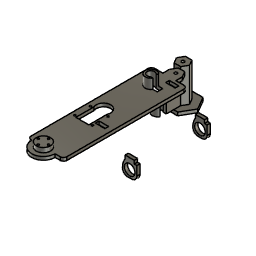
Arm Limb 2 Dynamixel v24 (Autodesk Fusion 360 design; units mm, degrees)
Autodesk Fusion 360 part; units mm, degrees
note: some values were not read from the file. Chosen so that the rebuilt part matches the saved one: which bodies a step acts on; which face or edge a step refers to. Set by a fixed rule: which sketch regions a step uses.
sketch "Sketch1" plane through (0, 0, 0) normal (0, 0, 1) x (1, 0, 0)
  circle A0 centre (25, 25) radius 1.5
  circle A1 centre (41, 25) radius 1.5
  circle A2 centre (33, 17) radius 1.5
  circle A3 centre (33, 33) radius 1.5
  circle A4 centre (33, 25) radius 18
  line L0 (15, 25) -> (51, 25)
  line L1 (51, 25) -> (51, 175)
  line L2 (51, 175) -> (15, 175)
  line L3 (15, 175) -> (15, 25)
  dimension "d1" = 3
  dimension "d2" = 3
  dimension "d3" = 3
  dimension "d4" = 3
  dimension "d5" = 36
  dimension "d6" = 150
  constraint horizontal L0
  constraint vertical L1
  constraint horizontal L2
  constraint vertical L3
  constraint coincident A4 L0.start
  measures "d1" diameter of A0
  measures "d2" diameter of A1
  measures "d3" diameter of A2
  measures "d4" diameter of A3
  measures "d5" distance of L0.start L0.end
  measures "d6" distance of L0.start L2.end
extrude "Extrude1" add sketch "Sketch1" along normal blind 5 contours A0 A1 A4 L0 | A0 A1 A4 L0 | A4 L1 L2 L3 makes body 1
sketch "Sketch4" plane through (0, 0, 0) normal (0, 0, 1) x (1, 0, 0)
  line L0 (50, 25) -> (70, 25)
  line L1 (70, 25) -> (70, 175)
  line L2 (70, 175) -> (50, 175)
  line L3 (50, 175) -> (50, 25)
  constraint horizontal L0
  constraint vertical L1
  constraint horizontal L2
  constraint vertical L3
extrude "Extrude3" add sketch "Sketch4" along normal blind 5 bodies 1
sketch "Sketch5" plane through (0, 0, 0) normal (0, 0, -1) x (1, 0, 0)
  line L0 (15, -175) -> (70, -175)
  line L1 (70, -175) -> (70, -25)
  line L2 (70, -25) -> (51, -25)
  arc A0 (51, -25) -> (15, -25) centre (33, -25) ccw
  line L3 (15, -25) -> (15, -175)
  circle A1 centre (33, -17) radius 1.5
  circle A2 centre (41, -25) radius 1.5
  circle A3 centre (25, -25) radius 1.5
  circle A4 centre (33, -33) radius 1.5
sketch "Sketch6" plane through (0, 0, 0) normal (0, 0, -1) x (1, 0, 0)
  line L0 (65.5, -170) -> (43.5, -170)
  line L1 (43.5, -170) -> (43.5, -165)
  line L2 (43.5, -165) -> (65.5, -165)
  line L3 (65.5, -165) -> (65.5, -170)
  line L4 (65.5, -62) -> (43.5, -62)
  line L5 (43.5, -62) -> (43.5, -57)
  line L6 (43.5, -57) -> (65.5, -57)
  line L7 (65.5, -57) -> (65.5, -62)
  dimension "d22" = 22
  dimension "d23" = 5
  dimension "d24" = 22
  dimension "d25" = 5
  constraint horizontal L0
  constraint vertical L1
  constraint horizontal L2
  constraint vertical L3
  constraint horizontal L4
  constraint vertical L5
  constraint horizontal L6
  constraint vertical L7
  measures "d22" distance of L0.start L0.end
  measures "d23" distance of L0.start L2.end
  measures "d24" distance of L4.start L4.end
  measures "d25" distance of L4.start L6.end
extrude "Extrude4" add sketch "Sketch6" along normal blind 22 bodies 1
sketch "Sketch7" plane through (0, 170, 0) normal (0, 1, 0) x (-1, 0, 0)
  line L0 (-43.5, 0) -> (-65.5, 0)
  line L1 (-65.5, 0) -> (-65.5, -22)
  line L2 (-65.5, -22) -> (-43.5, -22)
  line L3 (-43.5, -22) -> (-43.5, 0)
  circle A0 centre (-54.5, -11) radius 8.15
  dimension "d28" = 16.3
  measures "d28" diameter of A0
extrude "Extrude5" cut sketch "Sketch7" against normal blind 115 contours A0 bodies 1
fillet "Fillet1" radius 8 4 edges at (65.5, 167.5, -22) (43.5, 167.5, -22) (65.5, 59.5, -22) (43.5, 59.5, -22) on bodies 1
fillet "Fillet2" radius 5 3 edges at (70, 175, 2.5) (15, 175, 2.5) (70, 25, 2.5) on bodies 1
sketch "Sketch8" plane through (0, 0, 5) normal (0, 0, 1) x (-1, 0, 0)
  circle A0 centre (-33, -17) radius 1.5
  circle A1 centre (-41, -25) radius 1.5
  circle A2 centre (-25, -25) radius 1.5
  circle A3 centre (-33, -33) radius 1.5
  arc A4 (-65, -25) -> (-70, -30) centre (-65, -30) ccw
  line L0 (-70, -30) -> (-70, -170)
  arc A5 (-70, -170) -> (-65, -175) centre (-65, -170) ccw
  line L1 (-65, -175) -> (-20, -175)
  arc A6 (-20, -175) -> (-15, -170) centre (-20, -170) ccw
  line L2 (-15, -170) -> (-15, -25)
  arc A7 (-15, -25) -> (-51, -25) centre (-33, -25) ccw
  line L3 (-51, -25) -> (-65, -25)
  circle A8 centre (-39, -150) radius 5.75
  line L4 (-49.0301, -147.5429) -> (-43.0301, -147.5429)
  line L5 (-43.0301, -147.5429) -> (-43.0301, -152.5429)
  line L6 (-43.0301, -152.5429) -> (-49.0301, -152.5429)
  line L7 (-49.0301, -152.5429) -> (-49.0301, -147.5429)
  dimension "d35" = 11.5
  dimension "d42" = 6
  dimension "d43" = 5
  constraint horizontal L4
  constraint vertical L5
  constraint horizontal L6
  constraint vertical L7
  measures "d35" diameter of A8
  measures "d42" distance of L4.start L4.end
  measures "d43" distance of L4.start L6.end
extrude "Extrude6" cut sketch "Sketch8" against normal blind 5 contours A8 L4 L5 L6 | A8 L4 L5 L6 | A8 L4 L6 L7 bodies 1
sketch "Sketch9" plane through (0, 0, 5) normal (0, 0, 1) x (-1, 0, 0)
  arc A0 (-44.1572, -152.5429) -> (-44.1986, -147.5429) centre (-39, -150) ccw
  circle A1 centre (-33, -17) radius 1.5
  circle A2 centre (-41, -25) radius 1.5
  circle A3 centre (-25, -25) radius 1.5
  circle A4 centre (-33, -33) radius 1.5
  arc A5 (-65, -25) -> (-70, -30) centre (-65, -30) ccw
  line L0 (-70, -30) -> (-70, -170)
  arc A6 (-70, -170) -> (-65, -175) centre (-65, -170) ccw
  line L1 (-65, -175) -> (-20, -175)
  arc A7 (-20, -175) -> (-15, -170) centre (-20, -170) ccw
  line L2 (-15, -170) -> (-15, -25)
  arc A8 (-15, -25) -> (-51, -25) centre (-33, -25) ccw
  line L3 (-51, -25) -> (-65, -25)
  circle A9 centre (-39, -150) radius 8.6023
  line L4 (-49.0301, -147.5429) -> (-44.1986, -147.5429)
  line L5 (-44.1572, -152.5429) -> (-49.0301, -152.5429)
  line L6 (-49.0301, -152.5429) -> (-49.0301, -147.5429)
  constraint concentric A0 A9
extrude "Extrude7" add sketch "Sketch9" along normal blind 15 contours A0 A9 L4 L5 picked at (-45.6694, -153.7111) bodies 1
sketch "Sketch10" plane through (0, 0, 0) normal (0, 0, -1) x (1, 0, 0)
  line L0 (47.5, -170) -> (61.5, -170)
  line L1 (61.5, -170) -> (61.5, -165)
  line L2 (61.5, -165) -> (47.5, -165)
  line L3 (47.5, -165) -> (47.5, -170)
  line L4 (47.2, -170.3) -> (61.8, -170.3)
  line L5 (61.8, -170.3) -> (61.8, -164.7)
  line L6 (61.8, -164.7) -> (47.2, -164.7)
  line L7 (47.2, -164.7) -> (47.2, -170.3)
  line L8 (47.5, -62) -> (61.5, -62)
  line L9 (61.5, -62) -> (61.5, -57)
  line L10 (61.5, -57) -> (47.5, -57)
  line L11 (47.5, -57) -> (47.5, -62)
  line L12 (47.2, -62.3) -> (61.8, -62.3)
  line L13 (61.8, -62.3) -> (61.8, -56.7)
  line L14 (61.8, -56.7) -> (47.2, -56.7)
  line L15 (47.2, -56.7) -> (47.2, -62.3)
  dimension "d66" = 14.6
  dimension "d67" = 5.6
  constraint horizontal L0
  constraint vertical L1
  constraint horizontal L2
  constraint horizontal L4
  constraint vertical L5
  constraint horizontal L6
  constraint vertical L7
  constraint horizontal L8
  constraint vertical L9
  constraint horizontal L10
  constraint horizontal L12
  constraint vertical L13
  constraint horizontal L14
  constraint vertical L15
  measures "d66" distance of L5 L7
  measures "d67" distance of L4 L6
extrude "Extrude8" cut sketch "Sketch10" against normal blind 5 bodies 1
split "Split1" by plane through (0, 0, 0) normal (0, 0, 1) bodies 1 makes body 2 at (30.9251, 77.9076, 0) makes body 3 at (52.1667, 170, 1.6667) makes body 4 at (46.3905, 60.3333, -11.8115) makes body 5 at (52.1667, 60.3333, 5)
sketch "Sketch11" plane through (0, 0, 5) normal (0, 0, 1) x (-1, 0, 0)
  arc A0 (-45.7179, -152.5429) -> (-45.7439, -147.5429) centre (-37.5, -150) ccw
  line L0 (-45.7179, -152.5429) -> (-47.5301, -152.5429)
  line L1 (-47.5301, -152.5429) -> (-47.5301, -147.5429)
  line L2 (-47.5301, -147.5429) -> (-45.7439, -147.5429)
  circle A1 centre (-33, -17) radius 1.5
  circle A2 centre (-41, -25) radius 1.5
  circle A3 centre (-25, -25) radius 1.5
  circle A4 centre (-33, -33) radius 1.5
  arc A5 (-65, -25) -> (-70, -30) centre (-65, -30) ccw
  line L3 (-70, -30) -> (-70, -170)
  arc A6 (-70, -170) -> (-65, -175) centre (-65, -170) ccw
  line L4 (-65, -175) -> (-20, -175)
  arc A7 (-20, -175) -> (-15, -170) centre (-20, -170) ccw
  line L5 (-15, -170) -> (-15, -25)
  arc A8 (-15, -25) -> (-51, -25) centre (-33, -25) ccw
  line L6 (-51, -25) -> (-65, -25)
  circle A9 centre (-48, -75.3257) radius 1.5
  circle A10 centre (-21, -75.3257) radius 1.5
  circle A11 centre (-21, -51.3257) radius 1.5
  circle A12 centre (-48, -51.3257) radius 1.5
  line L7 (-47.2, -170.3) -> (-61.8, -170.3)
  line L8 (-61.8, -170.3) -> (-61.8, -164.7)
  line L9 (-61.8, -164.7) -> (-47.2, -164.7)
  line L10 (-47.2, -164.7) -> (-47.2, -170.3)
  line L11 (-47.2, -62.3) -> (-61.8, -62.3)
  line L12 (-61.8, -62.3) -> (-61.8, -56.7)
  line L13 (-61.8, -56.7) -> (-47.2, -56.7)
  line L14 (-47.2, -56.7) -> (-47.2, -62.3)
  circle A13 centre (-34.5, -81.8257) radius 11
  line L15 (-24.5, -49.3257) -> (-24.5, -77.2431)
  line L16 (-44.5, -49.3257) -> (-44.5, -77.2431)
  line L17 (-44.5, -49.3257) -> (-24.5, -49.3257)
  line L18 (-15, -175) -> (-15, -25)
  line L19 (-47.2, -170.3) -> (-61.8, -170.3)
  line L20 (-61.8, -170.3) -> (-61.8, -164.7)
  line L21 (-61.8, -164.7) -> (-47.2, -164.7)
  line L22 (-47.2, -164.7) -> (-47.2, -170.3)
  line L23 (-47.2, -62.3) -> (-61.8, -62.3)
  line L24 (-61.8, -62.3) -> (-61.8, -56.7)
  line L25 (-61.8, -56.7) -> (-47.2, -56.7)
  line L26 (-47.2, -56.7) -> (-47.2, -62.3)
  arc A14 (-47.2179, -152.5429) -> (-47.2439, -147.5429) centre (-39, -150) ccw
  line L27 (-47.2179, -152.5429) -> (-49.0301, -152.5429)
  line L28 (-49.0301, -152.5429) -> (-49.0301, -147.5429)
  line L29 (-49.0301, -147.5429) -> (-47.2439, -147.5429)
  circle A15 centre (-33, -17) radius 1.5
  circle A16 centre (-41, -25) radius 1.5
  circle A17 centre (-25, -25) radius 1.5
  circle A18 centre (-33, -33) radius 1.5
  arc A19 (-65, -25) -> (-70, -30) centre (-65, -30) ccw
  line L30 (-70, -30) -> (-70, -170)
  arc A20 (-70, -170) -> (-65, -175) centre (-65, -170) ccw
  line L31 (-65, -175) -> (-20, -175)
  arc A21 (-20, -175) -> (-15, -170) centre (-20, -170) ccw
  line L32 (-15, -170) -> (-15, -25)
  arc A22 (-15, -25) -> (-51, -25) centre (-33, -25) ccw
  line L33 (-51, -25) -> (-65, -25)
  dimension "d46" = 3
  dimension "d47" = 3
  dimension "d48" = 3
  dimension "d49" = 3
  dimension "d59" = 9.5
  dimension "d69" = 3.5
  dimension "d70" = 3.5
  dimension "d71" = 3.5
  dimension "d72" = 3.5
  constraint coincident A13 L15.end
  constraint vertical L15
  constraint coincident A13 L16.end
  constraint parallel L15 L16
  constraint perpendicular L16 L17
  measures "d46" diameter of A9
  measures "d47" diameter of A10
  measures "d48" diameter of A11
  measures "d49" diameter of A12
  measures "d59" distance of L5 L15
  measures "d69" distance of A10.centre L15
  measures "d70" distance of A9.centre L16
  measures "d71" distance of A12.centre L16
  measures "d72" distance of A11.centre L15
extrude "Extrude9" cut sketch "Sketch11" against normal blind 5 contours A9 | A10 | A11 | A12 | A13 | A13 L15 L16 L17 bodies 2
move_body "Move5" bodies 4 1 to x (1, 0, 0) y (0, 1, 0) z (0, 0, 1) at (0, 0, -25)
move_body "Move6" bodies 3 5 to x (1, 0, 0) y (0, 1, 0) z (0, 0, 1) at (0, 0, -25)
combine "Combine7" operation add target body 1 tool bodies 3
combine "Combine8" operation add target body 5 tool bodies 4
move_body "Move10" bodies 5 1 to x (1, 0, 0) y (0, 1, 0) z (0, 0, 1) at (40, 0, 0)
sketch "Sketch12" plane through (0, 0, 5) normal (0, 0, 1) x (-1, 0, 0)
  circle A0 centre (-48, -75.3257) radius 1.5
  circle A1 centre (-21, -75.3257) radius 1.5
  circle A2 centre (-48, -51.3257) radius 1.5
  circle A3 centre (-21, -51.3257) radius 1.5
  line L0 (-47.2, -170.3) -> (-61.8, -170.3)
  line L1 (-61.8, -170.3) -> (-61.8, -164.7)
  line L2 (-61.8, -164.7) -> (-47.2, -164.7)
  line L3 (-47.2, -164.7) -> (-47.2, -170.3)
  line L4 (-47.2, -62.3) -> (-61.8, -62.3)
  line L5 (-61.8, -62.3) -> (-61.8, -56.7)
  line L6 (-61.8, -56.7) -> (-47.2, -56.7)
  line L7 (-47.2, -56.7) -> (-47.2, -62.3)
  arc A4 (-47.2179, -152.5429) -> (-47.2439, -147.5429) centre (-39, -150) ccw
  line L8 (-47.2179, -152.5429) -> (-49.0301, -152.5429)
  line L9 (-49.0301, -152.5429) -> (-49.0301, -147.5429)
  line L10 (-49.0301, -147.5429) -> (-47.2439, -147.5429)
  circle A5 centre (-33, -17) radius 1.5
  circle A6 centre (-41, -25) radius 1.5
  circle A7 centre (-25, -25) radius 1.5
  circle A8 centre (-33, -33) radius 1.5
  arc A9 (-65, -25) -> (-70, -30) centre (-65, -30) ccw
  line L11 (-70, -30) -> (-70, -170)
  arc A10 (-70, -170) -> (-65, -175) centre (-65, -170) ccw
  line L12 (-65, -175) -> (-20, -175)
  arc A11 (-20, -175) -> (-15, -170) centre (-20, -170) ccw
  line L13 (-15, -170) -> (-15, -25)
  arc A12 (-15, -25) -> (-51, -25) centre (-33, -25) ccw
  line L14 (-51, -25) -> (-65, -25)
  circle A13 centre (-33, -25) radius 11
  line L15 (-44.5, -49.3257) -> (-24.5, -49.3257)
  line L16 (-24.5, -49.3257) -> (-24.5, -77.2431)
  line L17 (-44.5, -77.2431) -> (-44.5, -49.3257)
  arc A14 (-44.5, -77.2431) -> (-24.5, -77.2431) centre (-34.5, -81.8257) ccw
  dimension "d52" = 22
  constraint concentric A12 A13
  measures "d52" diameter of A13
extrude "Extrude10" add sketch "Sketch12" along normal blind 7 contours A13 bodies 2
move_body "Move7" bodies 2 to x (1, 0, 0) y (0, 1, 0) z (0, 0, 1) at (0, -45, 0)
split "Split2" by plane through (0, 0, 0) normal (0, 1, 0) bodies 2 makes body 6 at (60.2767, 81.6143, 0)
move_body "Move8" bodies 6 to x (1, 0, 0) y (0, 1, 0) z (0, 0, 1) at (0, 40, 0)
extrude "Extrude11" add 1 faces at (51.6667, 0, 1.6667) along direction (0, 1, 0) blind 40 on bodies 2 bodies 2 6
chamfer "Chamfer1" distance 4 angle 45 2 edges at (83.5, 59.5, -25) (83.5, 167.5, -25) on bodies 1 5
fillet "Fillet3" radius 25 2 edges at (83.5, 167.5, -29) (83.5, 59.5, -29) on bodies 1 5
sketch "Sketch16" plane through (0, -20, 0) normal (0, -1, 0) x (1, 0, 0)
  line L0 (65, 0) -> (65, 5)
  line L1 (65, 5) -> (51, 5)
  line L2 (51, 5) -> (51, 0)
  line L3 (51, 0) -> (65, 0)
extrude "Extrude12" cut 1 faces at (32.9626, -17.8319, 12) along direction (0, 0, -1) blind 30 on bodies 2 bodies 2
sketch "Sketch18" plane through (0, -20, 0) normal (0, -1, 0) x (1, 0, 0)
  line L0 (65, 0) -> (15, 0)
  line L1 (15, 0) -> (15, 5)
  line L2 (15, 5) -> (65, 5)
  line L3 (65, 5) -> (65, 0)
  constraint horizontal L0
  constraint vertical L1
  constraint horizontal L2
  constraint vertical L3
extrude "Extrude15" add sketch "Sketch18" against normal blind 20 bodies 2
extrude "Extrude16" cut sketch "Sketch18" along normal blind 23 bodies 2
sketch "Sketch19" plane through (0, 0, 5) normal (0, 0, 1) x (-1, 0, 0)
  arc A0 (-47.2179, -147.5429) -> (-47.2439, -142.5429) centre (-39, -145) ccw
  line L0 (-47.2179, -147.5429) -> (-49.0301, -147.5429)
  line L1 (-49.0301, -147.5429) -> (-49.0301, -142.5429)
  line L2 (-49.0301, -142.5429) -> (-47.2439, -142.5429)
  line L3 (-47.2, -57.3) -> (-61.8, -57.3)
  line L4 (-61.8, -57.3) -> (-61.8, -51.7)
  line L5 (-61.8, -51.7) -> (-47.2, -51.7)
  line L6 (-47.2, -51.7) -> (-47.2, -57.3)
  line L7 (-47.2, -165.3) -> (-61.8, -165.3)
  line L8 (-61.8, -165.3) -> (-61.8, -159.7)
  line L9 (-61.8, -159.7) -> (-47.2, -159.7)
  line L10 (-47.2, -159.7) -> (-47.2, -165.3)
  line L11 (-24.5, -44.3257) -> (-24.5, -72.2431)
  arc A1 (-44.5, -72.2431) -> (-24.5, -72.2431) centre (-34.5, -76.8257) ccw
  line L12 (-44.5, -72.2431) -> (-44.5, -44.3257)
  circle A2 centre (-21, -70.3257) radius 1.5
  circle A3 centre (-48, -70.3257) radius 1.5
  line L13 (-15, 20) -> (-65, 20)
  arc A4 (-65, 20) -> (-70, 15) centre (-65, 15) ccw
  line L14 (-70, 15) -> (-70, -165)
  arc A5 (-70, -165) -> (-65, -170) centre (-65, -165) ccw
  line L15 (-65, -170) -> (-20, -170)
  arc A6 (-20, -170) -> (-15, -165) centre (-20, -165) ccw
  line L16 (-15, -165) -> (-15, 20)
  line L17 (-39, -145) -> (-15, -145)
  line L18 (-15, -145) -> (-15, 20)
  line L19 (-15, 20) -> (-39, 20)
  line L20 (-39, 20) -> (-39, -145)
  circle A7 centre (-39, 20) radius 18
  circle A8 centre (-39, 20) radius 11
  circle A9 centre (-21, -46.3257) radius 1.5
  circle A10 centre (-48, -46.3257) radius 1.5
  line L21 (-44.5, -44.3257) -> (-24.5, -44.3257)
  dimension "d86" = 36
  dimension "d87" = 22
  constraint horizontal L17
  constraint vertical L18
  constraint horizontal L19
  constraint vertical L20
  constraint coincident L13.start L16.end
  constraint coincident A0.centre L17.start
  constraint coincident L19.end L20.start
  constraint concentric A7 A8
  measures "d86" diameter of A7
  measures "d87" diameter of A8
extrude "Extrude17" add sketch "Sketch19" along normal blind 7 contours L13 L19 L20 A8 | L13 L19 A8 | L13 L20 A8 bodies 2
extrude "Extrude18" add sketch "Sketch19" against normal blind 5 contours L13 L19 A7 A8 | L13 L19 A8 bodies 2
sketch "Sketch21" plane through (0, 0, 12) normal (0, 0, 1) x (-1, 0, 0)
  circle A0 centre (-39, 20) radius 11
  line L0 (-47, 12) -> (-31, 12)
  line L1 (-31, 12) -> (-31, 28)
  line L2 (-31, 28) -> (-47, 28)
  line L3 (-47, 28) -> (-47, 12)
  line L4 (-47, 12) -> (-31, 28) construction
  line L5 (-31, 12) -> (-47, 28) construction
  circle A1 centre (-39, 12) radius 1.5
  circle A2 centre (-47, 20) radius 1.5
  circle A3 centre (-39, 28) radius 1.5
  circle A4 centre (-31, 20) radius 1.5
  point P0 (-39, 20)
  dimension "d94" = 16
  dimension "d95" = 16
  dimension "d96" = 3
  dimension "d97" = 3
  dimension "d98" = 3
  dimension "d99" = 3
  constraint horizontal L0
  constraint perpendicular L0 L1
  constraint parallel L0 L2
  constraint parallel L1 L3
  constraint coincident L4 P0
  constraint coincident L5 P0
  constraint coincident P0 A0.centre
  constraint midpoint L0 A1.centre
  constraint midpoint L3 A2.centre
  constraint midpoint L2 A3.centre
  constraint midpoint L1 A4.centre
  measures "d94" distance of L1.end L2.end
  measures "d95" distance of L0.end L1.end
  measures "d96" diameter of A1
  measures "d97" diameter of A2
  measures "d98" diameter of A3
  measures "d99" diameter of A4
extrude "Extrude19" cut sketch "Sketch21" against normal blind 20 contours L1 A4 | L1 A4 | L2 A3 | L2 A3 | L0 A1 | L0 A1 | L3 A2 | L3 A2 bodies 2
fillet "Fillet4" radius 5 1 edges at (15, -20, 2.5) on bodies 2
extrude "Extrude20" cut 1 faces at (49.0301, 145.8762, 3.3333) along direction (1, 0, 0) blind 2 on bodies 2 bodies 2
sketch "Sketch23" plane through (0, 170, 0) normal (0, 1, 0) x (-1, 0, 0)
  line L0 (-20, 0) -> (-20, 5)
  line L1 (-20, 5) -> (-65, 5)
  line L2 (-65, 5) -> (-65, 0)
  line L3 (-65, 0) -> (-20, 0)
  line L4 (-32.5, 0) -> (-52.5, 0)
  line L5 (-52.5, 0) -> (-52.5, 5)
  line L6 (-52.5, 5) -> (-32.5, 5)
  line L7 (-32.5, 5) -> (-32.5, 0)
  line L8 (-32.5, 0) -> (-52.5, 5) construction
  line L9 (-52.5, 0) -> (-32.5, 5) construction
  point P0 (-42.5, 2.5)
  constraint horizontal L4
  constraint perpendicular L4 L5
  constraint parallel L4 L6
  constraint parallel L5 L7
  constraint coincident L8 P0
  constraint coincident L9 P0
  constraint coincident L3 L4.start
extrude "Extrude23" add sketch "Sketch23" along normal blind 20 contours L1 L3 L4 L5 L6 L7 bodies 2
sketch "Sketch24" plane through (0, 0, 0) normal (0, 0, -1) x (1, 0, 0)
  line L0 (51.0301, -147.5429) -> (44.1572, -147.5429)
  arc A0 (44.1986, -142.5429) -> (44.1572, -147.5429) centre (39, -145) ccw
  line L1 (44.1986, -142.5429) -> (51.0301, -142.5429)
  line L2 (51.0301, -142.5429) -> (51.0301, -147.5429)
  arc A1 (20, 20) -> (15, 15) centre (20, 15) ccw
  line L3 (15, 15) -> (15, -165)
  arc A2 (15, -165) -> (20, -170) centre (20, -165) ccw
  line L4 (20, -170) -> (32.5, -170)
  line L5 (32.5, -170) -> (32.5, -190)
  line L6 (32.5, -190) -> (52.5, -190)
  line L7 (52.5, -190) -> (52.5, -170)
  line L8 (52.5, -170) -> (65, -170)
  arc A3 (65, -170) -> (70, -165) centre (65, -165) ccw
  line L9 (70, -165) -> (70, 15)
  arc A4 (70, 15) -> (65, 20) centre (65, 15) ccw
  line L10 (65, 20) -> (57, 20)
  arc A5 (57, 20) -> (21, 20) centre (39, 20) ccw
  line L11 (21, 20) -> (20, 20)
  circle A6 centre (39, 28) radius 1.5
  circle A7 centre (31, 20) radius 1.5
  circle A8 centre (47, 20) radius 1.5
  circle A9 centre (39, 12) radius 1.5
  circle A10 centre (48, -70.3257) radius 1.5
  circle A11 centre (21, -70.3257) radius 1.5
  line L12 (24.5, -72.2431) -> (24.5, -44.3257)
  line L13 (24.5, -44.3257) -> (44.5, -44.3257)
  line L14 (44.5, -44.3257) -> (44.5, -72.2431)
  arc A12 (24.5, -72.2431) -> (44.5, -72.2431) centre (34.5, -76.8257) ccw
  circle A13 centre (48, -46.3257) radius 1.5
  circle A14 centre (21, -46.3257) radius 1.5
  line L15 (47.2, -165.3) -> (47.2, -159.7)
  line L16 (47.2, -159.7) -> (61.8, -159.7)
  line L17 (61.8, -159.7) -> (61.8, -165.3)
  line L18 (61.8, -165.3) -> (47.2, -165.3)
  line L19 (47.2, -57.3) -> (47.2, -51.7)
  line L20 (47.2, -51.7) -> (61.8, -51.7)
  line L21 (61.8, -51.7) -> (61.8, -57.3)
  line L22 (61.8, -57.3) -> (47.2, -57.3)
  line L23 (32.5, -180) -> (37.5, -188.6603)
  line L24 (37.5, -188.6603) -> (47.5, -188.6603)
  line L25 (47.5, -188.6603) -> (52.5, -180)
  line L26 (52.5, -180) -> (47.5, -171.3397)
  line L27 (47.5, -171.3397) -> (37.5, -171.3397)
  line L28 (37.5, -171.3397) -> (32.5, -180)
  point P0 (42.5, -180)
  constraint midpoint L5 L23.start
extrude "Extrude24" cut sketch "Sketch24" against normal blind 5 contours L5 L6 L7 L23 L24 L25 bodies 2
extrude "Extrude25" add sketch "Sketch24" along normal blind 52 contours L23 L24 L25 L26 L27 L28 bodies 2
sketch "Sketch25" plane through (0, 0, -52) normal (0, 0, -1) x (1, 0, 0)
  line L0 (37.5, -171.3397) -> (32.5, -180)
  line L1 (32.5, -180) -> (37.5, -188.6603)
  line L2 (37.5, -188.6603) -> (47.5, -188.6603)
  line L3 (47.5, -188.6603) -> (52.5, -180)
  line L4 (52.5, -180) -> (47.5, -171.3397)
  line L5 (47.5, -171.3397) -> (37.5, -171.3397)
  line L6 (65, -180) -> (53.75, -160.5144)
  line L7 (53.75, -160.5144) -> (31.25, -160.5144)
  line L8 (31.25, -160.5144) -> (20, -180)
  line L9 (20, -180) -> (31.25, -199.4856)
  line L10 (31.25, -199.4856) -> (53.75, -199.4856)
  line L11 (53.75, -199.4856) -> (65, -180)
  point P0 (42.5, -180)
extrude "Extrude26" add sketch "Sketch25" along normal blind 5 contours L0 L1 L2 L3 L4 L5 | L6 L7 L8 L9 L10 L11 bodies 2
sketch "Sketch26" plane through (0, 0, 5) normal (0, 0, 1) x (-1, 0, 0)
  circle A0 centre (-48, -70.3257) radius 1.5
  circle A1 centre (-21, -70.3257) radius 1.5
  line L0 (-24.5, -44.3257) -> (-24.5, -72.2431)
  arc A2 (-44.5, -72.2431) -> (-24.5, -72.2431) centre (-34.5, -76.8257) ccw
  line L1 (-44.5, -72.2431) -> (-44.5, -44.3257)
  line L2 (-44.5, -44.3257) -> (-24.5, -44.3257)
  circle A3 centre (-48, -46.3257) radius 1.5
  circle A4 centre (-21, -46.3257) radius 1.5
  line L3 (-47.2, -165.3) -> (-61.8, -165.3)
  line L4 (-61.8, -165.3) -> (-61.8, -159.7)
  line L5 (-61.8, -159.7) -> (-47.2, -159.7)
  line L6 (-47.2, -159.7) -> (-47.2, -165.3)
  line L7 (-47.2, -57.3) -> (-61.8, -57.3)
  line L8 (-61.8, -57.3) -> (-61.8, -51.7)
  line L9 (-61.8, -51.7) -> (-47.2, -51.7)
  line L10 (-47.2, -51.7) -> (-47.2, -57.3)
  line L11 (-47.2179, -147.5429) -> (-51.0301, -147.5429)
  line L12 (-51.0301, -147.5429) -> (-51.0301, -142.5429)
  line L13 (-51.0301, -142.5429) -> (-47.2439, -142.5429)
  arc A5 (-47.2179, -147.5429) -> (-47.2439, -142.5429) centre (-39, -145) ccw
  line L14 (-52.5, -180) -> (-47.5, -188.6603)
  line L15 (-47.5, -188.6603) -> (-37.5, -188.6603)
  line L16 (-37.5, -188.6603) -> (-32.5, -180)
  line L17 (-32.5, -180) -> (-32.5, -170)
  line L18 (-32.5, -170) -> (-20, -170)
  arc A6 (-20, -170) -> (-15, -165) centre (-20, -165) ccw
  line L19 (-15, -165) -> (-15, 15)
  arc A7 (-15, 15) -> (-20, 20) centre (-20, 15) ccw
  line L20 (-20, 20) -> (-21, 20)
  arc A8 (-21, 20) -> (-57, 20) centre (-39, 20) ccw
  line L21 (-57, 20) -> (-65, 20)
  arc A9 (-65, 20) -> (-70, 15) centre (-65, 15) ccw
  line L22 (-70, 15) -> (-70, -165)
  arc A10 (-70, -165) -> (-65, -170) centre (-65, -165) ccw
  line L23 (-65, -170) -> (-52.5, -170)
  line L24 (-52.5, -170) -> (-52.5, -180)
  circle A11 centre (-39, 20) radius 11
  circle A12 centre (-42.5, -180) radius 2.25
  dimension "d121" = 4.5
  measures "d121" diameter of A12
extrude "Extrude27" cut sketch "Sketch26" against normal blind 16 contours A12 bodies 2
extrude "Extrude28" add 1 faces at (45.6682, 148.7131, 20) along direction (0, 0, -1) blind 65 on bodies 2 bodies 2
sketch "Sketch29" plane through (0, 0, 0) normal (0, 0, -1) x (1, 0, 0)
  line L0 (47.2, -57.3) -> (47.2, -51.7)
  line L1 (47.2, -51.7) -> (61.8, -51.7)
  line L2 (61.8, -51.7) -> (61.8, -57.3)
  line L3 (61.8, -57.3) -> (47.2, -57.3)
  line L4 (47.2, -165.3) -> (47.2, -159.7)
  line L5 (47.2, -159.7) -> (61.8, -159.7)
  line L6 (61.8, -159.7) -> (61.8, -165.3)
  line L7 (61.8, -165.3) -> (47.2, -165.3)
  circle A0 centre (21, -46.3257) radius 1.5
  circle A1 centre (48, -46.3257) radius 1.5
  line L8 (24.5, -72.2431) -> (24.5, -44.3257)
  line L9 (24.5, -44.3257) -> (44.5, -44.3257)
  line L10 (44.5, -44.3257) -> (44.5, -72.2431)
  arc A2 (24.5, -72.2431) -> (44.5, -72.2431) centre (34.5, -76.8257) ccw
  circle A3 centre (21, -70.3257) radius 1.5
  circle A4 centre (48, -70.3257) radius 1.5
  circle A5 centre (39, 12) radius 1.5
  circle A6 centre (47, 20) radius 1.5
  circle A7 centre (31, 20) radius 1.5
  circle A8 centre (39, 28) radius 1.5
  arc A9 (47.2439, -142.5429) -> (47.2179, -147.5429) centre (39, -145) ccw
  line L11 (47.2439, -142.5429) -> (51.0301, -142.5429)
  line L12 (51.0301, -142.5429) -> (51.0301, -147.5429)
  line L13 (51.0301, -147.5429) -> (47.2179, -147.5429)
  line L14 (47.5, -171.3397) -> (52.5, -180)
  line L15 (52.5, -180) -> (52.5, -170)
  line L16 (52.5, -170) -> (65, -170)
  arc A10 (65, -170) -> (70, -165) centre (65, -165) ccw
  line L17 (70, -165) -> (70, 15)
  arc A11 (70, 15) -> (65, 20) centre (65, 15) ccw
  line L18 (65, 20) -> (57, 20)
  arc A12 (57, 20) -> (21, 20) centre (39, 20) ccw
  line L19 (21, 20) -> (20, 20)
  arc A13 (20, 20) -> (15, 15) centre (20, 15) ccw
  line L20 (15, 15) -> (15, -165)
  arc A14 (15, -165) -> (20, -170) centre (20, -165) ccw
  line L21 (20, -170) -> (32.5, -170)
  line L22 (32.5, -170) -> (32.5, -180)
  line L23 (32.5, -180) -> (37.5, -171.3397)
  line L24 (37.5, -171.3397) -> (47.5, -171.3397)
  circle A15 centre (39, -145) radius 8.6023
  circle A16 centre (39, -145) radius 5.7423
  constraint concentric A9 A15
  constraint concentric A9 A16
extrude "Extrude29" cut sketch "Sketch29" along normal blind 25 contours A9 A15 bodies 2 makes body 7 at (47.111, 142.1344, -38.3333)
move_body "Move11" bodies 7 to x (1, 0, 0) y (0, 1, 0) z (0, 0, 1) at (0, 0, -7)
sketch "Sketch30" plane through (0, 171.3397, 0) normal (0, -1, 0) x (1, 0, 0)
  line L0 (47.5, 0) -> (37.5, 0)
  line L1 (37.5, 0) -> (37.5, -52)
  line L2 (37.5, -52) -> (47.5, -52)
  line L3 (47.5, -52) -> (47.5, 0)
  line L4 (37.5, -32) -> (47.5, -32)
  line L5 (47.5, -32) -> (47.5, -52)
  line L6 (47.5, -52) -> (37.5, -52)
  line L7 (37.5, -52) -> (37.5, -32)
  constraint horizontal L4
  constraint vertical L5
  constraint horizontal L6
  constraint vertical L7
  constraint coincident L2.end L3.start
  constraint coincident L1 L4.start
extrude "Extrude30" add sketch "Sketch30" along normal blind 24 contours L1 L2 L3 L4 L5 L6 L7 bodies 2 7
extrude "Extrude31" cut sketch "Sketch29" along normal blind 50 contours A16 bodies 2
split "Split3" by plane through (0, 0, 0) normal (0, 0, 1) bodies 2 makes body 8 at (52.6946, 6.3874, 0)
move_body "Move9" bodies 2 to x (1, 0, 0) y (0, 1, 0) z (0, 0, 1) at (-15, 25.9808, 0)
sketch "Sketch31" plane through (0, 0, 5) normal (0, 0, 1) x (-1, 0, 0)
  circle A0 centre (-42.5, -180) radius 2.25
  circle A1 centre (-48, -70.3257) radius 1.5
  circle A2 centre (-21, -70.3257) radius 1.5
  line L0 (-24.5, -44.3257) -> (-24.5, -72.2431)
  arc A3 (-44.5, -72.2431) -> (-24.5, -72.2431) centre (-34.5, -76.8257) ccw
  line L1 (-44.5, -72.2431) -> (-44.5, -44.3257)
  line L2 (-44.5, -44.3257) -> (-24.5, -44.3257)
  circle A4 centre (-48, -46.3257) radius 1.5
  circle A5 centre (-21, -46.3257) radius 1.5
  line L3 (-47.2, -165.3) -> (-61.8, -165.3)
  line L4 (-61.8, -165.3) -> (-61.8, -159.7)
  line L5 (-61.8, -159.7) -> (-47.2, -159.7)
  line L6 (-47.2, -159.7) -> (-47.2, -165.3)
  line L7 (-47.2, -57.3) -> (-61.8, -57.3)
  line L8 (-61.8, -57.3) -> (-61.8, -51.7)
  line L9 (-61.8, -51.7) -> (-47.2, -51.7)
  line L10 (-47.2, -51.7) -> (-47.2, -57.3)
  line L11 (-47.2179, -147.5429) -> (-51.0301, -147.5429)
  line L12 (-51.0301, -147.5429) -> (-51.0301, -142.5429)
  line L13 (-51.0301, -142.5429) -> (-47.2439, -142.5429)
  arc A6 (-47.2179, -147.5429) -> (-47.2439, -142.5429) centre (-39, -145) ccw
  line L14 (-52.5, -180) -> (-47.5, -188.6603)
  line L15 (-47.5, -188.6603) -> (-37.5, -188.6603)
  line L16 (-37.5, -188.6603) -> (-32.5, -180)
  line L17 (-32.5, -180) -> (-32.5, -170)
  line L18 (-32.5, -170) -> (-20, -170)
  arc A7 (-20, -170) -> (-15, -165) centre (-20, -165) ccw
  line L19 (-15, -165) -> (-15, 15)
  arc A8 (-15, 15) -> (-20, 20) centre (-20, 15) ccw
  line L20 (-20, 20) -> (-21, 20)
  arc A9 (-21, 20) -> (-57, 20) centre (-39, 20) ccw
  line L21 (-57, 20) -> (-65, 20)
  arc A10 (-65, 20) -> (-70, 15) centre (-65, 15) ccw
  line L22 (-70, 15) -> (-70, -165)
  arc A11 (-70, -165) -> (-65, -170) centre (-65, -165) ccw
  line L23 (-65, -170) -> (-52.5, -170)
  line L24 (-52.5, -170) -> (-52.5, -180)
  circle A12 centre (-39, 20) radius 11
  line L25 (-42.7923, -140.75) -> (-53, -140.75)
  line L26 (-53, -140.75) -> (-53, -149.25)
  line L27 (-53, -149.25) -> (-42.7923, -149.25)
  line L28 (-42.7923, -149.25) -> (-42.7923, -140.75)
  line L29 (-42.7923, -140.75) -> (-53, -149.25) construction
  line L30 (-53, -140.75) -> (-42.7923, -149.25) construction
  point P0 (-47.8961, -145)
  point P1 (-47.8961, -145)
  dimension "d132" = 8.5
  constraint horizontal L25
  constraint perpendicular L25 L26
  constraint parallel L25 L27
  constraint parallel L26 L28
  constraint coincident L29 P1
  constraint coincident L30 P1
  constraint coincident P1 P0
  measures "d132" distance of L25.end L26.end
extrude "Extrude32" cut sketch "Sketch31" along normal blind 15 and the other way blind 20 contours L11 L12 L13 A6 L25 L26 L27 | L11 L12 L13 A6 L25 L27 L28 bodies 8
sketch "Sketch32" plane through (0, 0, -52) normal (0, 0, -1) x (1, 0, 0)
  line L0 (22.5, -179.4513) -> (22.5, -186.4952)
  line L1 (22.5, -186.4952) -> (32.5, -186.4952)
  line L2 (32.5, -186.4952) -> (32.5, -173.3205)
  line L3 (32.5, -173.3205) -> (22.5, -173.3205)
  line L4 (22.5, -173.3205) -> (22.5, -176.5317)
  arc A0 (29.1986, -168.5236) -> (22.5, -176.5317) centre (24, -170.9808) ccw
  line L5 (29.1986, -168.5236) -> (32.2439, -168.5236)
  arc A1 (32.2439, -168.5236) -> (22.5, -179.4513) centre (24, -170.9808) ccw
  circle A2 centre (24, -170.9808) radius 5.75
  line L6 (37, -166.75) -> (27, -166.75)
  line L7 (27, -166.75) -> (27, -175.25)
  line L8 (27, -175.25) -> (37, -175.25)
  line L9 (37, -175.25) -> (37, -166.75)
  line L10 (37, -166.75) -> (27, -175.25) construction
  line L11 (27, -166.75) -> (37, -175.25) construction
  point P0 (32, -171)
  point P1 (32, -171)
  dimension "d140" = 8.5
  constraint concentric A0 A2
  constraint coincident A0.start A2
  constraint horizontal L6
  constraint perpendicular L6 L7
  constraint parallel L6 L8
  constraint parallel L7 L9
  constraint coincident L10 P1
  constraint coincident L11 P1
  constraint coincident P1 P0
  measures "d140" distance of L6.end L7.end
extrude "Extrude33" cut sketch "Sketch32" against normal blind 25 contours L2 L3 L5 A1 A2 L6 L8 L9 | A0 L5 A1 A2 L6 | L3 L4 A0 A2 L6 L7 | L3 A0 A2 L6 L7 | L2 L3 A2 L8 | L3 L4 A2 L7 L8 | L3 A2 L7 L8 bodies 2
equation "d59 = 8 mm + 1.5 mm"
